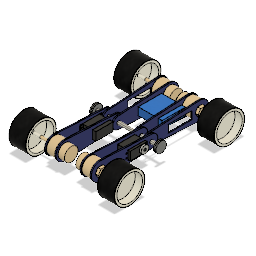
car v16 (Autodesk Fusion 360 design; units mm, degrees)
Autodesk Fusion 360 part; units mm, degrees
sketch "Sketch1" plane through (0, 0, 0) normal (0, 0, 1) x (1, 0, 0) in component "far_leg"
  circle A0 centre (0, 0) radius 6.5
  line L0 (0, 0) -> (120, 0)
  circle A1 centre (120, 0) radius 4
  line L1 (1.225, 20.9642) -> (120.8167, 13.9762)
  line L2 (1.225, -20.9642) -> (120.8167, -13.9762)
  line L3 (19, 0) -> (19, 9)
  line L4 (19, 9) -> (74, 9)
  line L5 (74, 9) -> (74, -9)
  line L6 (74, -9) -> (19, -9)
  line L7 (19, -9) -> (19, 0)
  arc A2 (1.225, 20.9642) -> (1.225, -20.9642) centre (0, 0) ccw
  arc A3 (120.8167, -13.9762) -> (120.8167, 13.9762) centre (120, 0) ccw
  dimension "d1" = 13
  dimension "d2" = 120
  dimension "d3" = 8
  dimension "d4" = 42
  dimension "d5" = 28
  dimension "d183" = 19
  dimension "d184" = 9
  dimension "d186" = 55
  dimension "d187" = 18
  dimension "d188" = 55
  dimension "d272" = 9
  constraint coincident A0.centre L0.start
  constraint horizontal L0
  constraint coincident L0.end A1.centre
  constraint concentric A1 A3
  constraint tangent L1 A3
  constraint tangent L2 A3
  constraint tangent L1 A2
  constraint tangent L2 A2
  constraint perpendicular L0 L3
  constraint perpendicular L3 L4
  constraint perpendicular L0 L5
  constraint perpendicular L5 L6
  measures "d1" diameter of A0
  measures "d2" distance of A0.centre L0.end
  measures "d3" diameter of A1
  measures "d4" diameter of A2
  measures "d5" diameter of A3
  measures "d183" distance of A0.centre L3.start
  measures "d184" distance of L3.start L3.end
  measures "d186" distance of L3.end L4.end
  measures "d187" distance of L4.end L5.end
  measures "d188" distance of L5.end L6.end
  measures "d272" distance of L0 L4
extrude "Extrude1" add sketch "Sketch1" along normal blind 3 makes body 1 in component "far_leg"
sketch "Sketch1 (2)" plane through (0, 0, 0) normal (0, 0, 1) x (1, 0, 0) in component "motor"
  circle A0 centre (0, 0) radius 16
  dimension "d37" = 32
  constraint coincident A0.centre origin
  measures "d37" diameter of A0
extrude "Extrude1'" add sketch "Sketch1 (2)" along normal blind 18 separate body makes body 2 in component "motor"
sketch "Sketch2" plane through (0, 0, 18) normal (0, 0, 1) x (1, 0, 0) in component "motor"
  circle A0 centre (0, 0) radius 16
  circle A1 centre (0, 0) radius 19
  dimension "d40" = 38
  constraint coincident A0.centre A1.centre
  measures "d40" diameter of A1
extrude "Extrude2" add sketch "Sketch2" along normal blind 21 contours A0 | A1 bodies 2 in component "motor"
sketch "Sketch3" plane through (0, 0, 39) normal (0, 0, 1) x (1, 0, 0) in component "motor"
  circle A0 centre (0, 0) radius 19
  line L0 (5.75, -9.9593) -> (11.5, 0)
  line L1 (11.5, 0) -> (5.75, 9.9593)
  line L2 (5.75, 9.9593) -> (-5.75, 9.9593)
  line L3 (-5.75, 9.9593) -> (-11.5, 0)
  line L4 (-11.5, 0) -> (-5.75, -9.9593)
  line L5 (-5.75, -9.9593) -> (5.75, -9.9593)
  line L6 (0, 0) -> (29.7634, 0) construction
  dimension "d43" = 11.5
  constraint coincident A0.centre L6.start
  constraint horizontal L6
  constraint parallel L2 L6
  measures "d43" distance of L0.start A0.centre
extrude "Extrude3" add sketch "Sketch3" along normal blind 10 and the other way blind -3 separate body contours L0 L1 L2 L3 L4 L5 makes body 3 in component "motor"
sketch "Sketch4" plane through (0, 0, 49) normal (0, 0, 1) x (1, 0, 0) in component "motor"
  line L0 (-5.75, -9.9593) -> (5.75, -9.9593)
  line L1 (5.75, -9.9593) -> (11.5, 0)
  line L2 (11.5, 0) -> (5.75, 9.9593)
  line L3 (5.75, 9.9593) -> (-5.75, 9.9593)
  line L4 (-5.75, 9.9593) -> (-11.5, 0)
  line L5 (-11.5, 0) -> (-5.75, -9.9593)
  circle A0 centre (0, 0) radius 3
  dimension "d46" = 6
  constraint coincident A0.centre origin
  measures "d46" diameter of A0
extrude "Extrude4" add sketch "Sketch4" along normal blind 22 and the other way up to surface (10 mm away) contours A0 bodies 3 2 in component "motor"
sketch "Sketch1 (3)" plane through (0, 0, 0) normal (0, 0, 1) x (1, 0, 0) in component "wheel"
  circle A0 centre (0, 0) radius 35
  circle A1 centre (0, 0) radius 30
  dimension "d49" = 70
  dimension "d50" = 60
  constraint coincident A0.centre A1.centre
  measures "d49" diameter of A0
  measures "d50" diameter of A1
extrude "Extrude1''" add sketch "Sketch1 (3)" along normal mid plane 40 separate body makes body 4 in component "wheel"
sketch "Sketch2 (2)" plane through (0, 0, 0) normal (0, 0, 1) x (1, 0, 0) in component "wheel"
  circle A0 centre (0, 0) radius 30
  dimension "d53" = 60
  constraint coincident A0.centre origin
  measures "d53" diameter of A0
extrude "Extrude2'" add sketch "Sketch2 (2)" along normal mid plane 6 bodies 4 in component "wheel"
sketch "Sketch3 (2)" plane through (0, 0, -3) normal (0, 0, -1) x (-1, 0, 0) in component "wheel"
  circle A0 centre (0, 0) radius 30
  circle A1 centre (0, 0) radius 3
  dimension "d56" = 6
  constraint coincident A0.centre A1.centre
  measures "d56" diameter of A1
extrude "Extrude3'" add sketch "Sketch3 (2)" along normal blind 17 contours A1 bodies 4 in component "wheel"
sketch "Sketch1 (4)" plane through (0, 0, 0) normal (0, 0, 1) x (1, 0, 0) in component "tyre"
  circle A0 centre (0, 0) radius 35
  circle A1 centre (0, 0) radius 36
  dimension "d68" = 70
  dimension "d69" = 72
  constraint coincident A0.centre A1.centre
  constraint concentric A0 A1
  measures "d68" diameter of A0
  measures "d69" diameter of A1
extrude "Extrude1'''" add sketch "Sketch1 (4)" along normal mid plane 40 separate body makes body 5 in component "tyre"
move_body "Move1" bodies 4 to x (0, 0, 1) y (0, 1, 0) z (-1, 0, 0) at (44, 0, -196) in component "wheel"
move_body "Move1'" bodies 3 to x (0, 0, 1) y (0, 1, 0) z (-1, 0, 0) at (135, 0, -105) in component "motor"
move_body "Move1''" bodies 1 to x (0, 0, 1) y (0, 1, 0) z (-1, 0, 0) at (96, 0, -144) in component "far_leg"
move_body "Move1'''" bodies 5 to x (0, 0, 1) y (0, 1, 0) z (-1, 0, 0) at (44, 0, -196) in component "tyre"
sketch "Sketch1 (5)" plane through (0, 0, 0) normal (1, 0, 0) x (0, 0, -1) in component "axle"
  circle A0 centre (0, 0) radius 4
  dimension "d156" = 8
  constraint coincident A0.centre origin
  measures "d156" diameter of A0
extrude "Extrude1''''" add sketch "Sketch1 (5)" along normal blind 150 separate body makes body 6 in component "axle"
sketch "Sketch1 (6)" plane through (0, 0, 0) normal (1, 0, 0) x (0, 0, -1) in component "front_far_leg"
  circle A0 centre (0, 0) radius 4
  line L0 (0, 0) -> (-132.6267, 0) construction
  line L1 (0, 0) -> (0, 16.3072) construction
  line L2 (0, 0) -> (0, -19.0636) construction
  circle A1 centre (-120, 0) radius 6.5
  line L3 (-15, 10) -> (-55, 10)
  line L4 (-55, 10) -> (-55, -10)
  line L5 (-55, -10) -> (-15, -10)
  line L6 (-15, -10) -> (-15, 10)
  line L7 (0, 15) -> (-118.9467, 20.9736)
  line L8 (0, -15) -> (-118.9467, -20.9736)
  arc A2 (-118.9467, 20.9736) -> (-118.9467, -20.9736) centre (-120, 0) ccw
  arc A3 (0, -15) -> (0, 15) centre (0, 0) ccw
  line L9 (-15, 5) -> (-11, 5) construction
  line L10 (-15, -5) -> (-11, -5) construction
  line L11 (-55, 5) -> (-59, 5) construction
  line L12 (-55, -5) -> (-59, -5) construction
  circle A4 centre (-11, 5) radius 1.5
  circle A5 centre (-11, -5) radius 1.5
  circle A6 centre (-59, 5) radius 1.5
  circle A7 centre (-59, -5) radius 1.5
  dimension "d288" = 8
  dimension "d289" = 30
  dimension "d290" = 13
  dimension "d291" = 42
  dimension "d292" = 120
  dimension "d293" = 40
  dimension "d294" = 20
  dimension "d295" = 10
  dimension "d296" = 15
  dimension "d398" = 4
  dimension "d399" = 4
  dimension "d400" = 4
  dimension "d401" = 4
  dimension "d402" = 5
  dimension "d403" = 5
  dimension "d404" = 5
  dimension "d405" = 5
  dimension "d406" = 3
  dimension "d407" = 3
  dimension "d408" = 3
  dimension "d409" = 3
  constraint coincident A0.centre L0.start
  constraint concentric A0 A3
  constraint horizontal L0
  constraint perpendicular L0 L1
  constraint perpendicular L0 L2
  constraint coincident L0 A1.centre
  constraint concentric A1 A2
  constraint horizontal L3
  constraint vertical L4
  constraint horizontal L5
  constraint vertical L6
  constraint coincident L1 L7.start
  constraint tangent L7 A2
  constraint coincident L2 L8.start
  constraint tangent L8 A2
  constraint coincident L6 L9.start
  constraint perpendicular L6 L9
  constraint coincident L6 L10.start
  constraint perpendicular L6 L10
  constraint coincident L4 L11.start
  constraint perpendicular L4 L11
  constraint coincident L4 L12.start
  constraint perpendicular L4 L12
  constraint coincident L9.end A4.centre
  constraint coincident L10.end A5.centre
  constraint coincident L11.end A6.centre
  constraint coincident L12.end A7.centre
  measures "d288" diameter of A0
  measures "d289" diameter of A3
  measures "d290" diameter of A1
  measures "d291" diameter of A2
  measures "d292" distance of A0.centre A1.centre
  measures "d293" distance of L3.start L3.end
  measures "d294" distance of L3.start L5.end
  measures "d295" distance of L0 L3
  measures "d296" distance of L2 L6
  measures "d398" distance of L9.start L9.end
  measures "d399" distance of L10.start L10.end
  measures "d400" distance of L11.start L11.end
  measures "d401" distance of L12.start L12.end
  measures "d402" distance of L0 L9
  measures "d403" distance of L0 L10
  measures "d404" distance of L0 L11
  measures "d405" distance of L0 L12
  measures "d406" diameter of A4
  measures "d407" diameter of A5
  measures "d408" diameter of A6
  measures "d409" diameter of A7
extrude "Extrude1'''''" add sketch "Sketch1 (6)" along normal blind 3 separate body makes body 7 in component "front_far_leg"
sketch "Sketch1 (7)" plane through (0, 0, 0) normal (1, 0, 0) x (0, 0, -1) in component "front_mid_leg"
  line L0 (-15, -10) -> (-15, 10)
  line L1 (0, 0) -> (-150, 0) construction
  circle A0 centre (-120, 0) radius 16
  line L2 (-55, -10) -> (-15, -10)
  line L3 (0, 0) -> (0, 25.1671) construction
  line L4 (-55, 10) -> (-55, -10)
  line L5 (0, 15) -> (-118.9467, 20.9736)
  line L6 (-15, 10) -> (-55, 10)
  line L7 (0, -15) -> (-118.9467, -20.9736)
  circle A1 centre (0, 0) radius 4
  line L8 (0, 0) -> (0, 72.997) construction
  arc A2 (0, -15) -> (0, 15) centre (0, 0) ccw
  arc A3 (-118.9467, 20.9736) -> (-118.9467, -20.9736) centre (-120, 0) ccw
  dimension "d309" = 8
  dimension "d310" = 30
  dimension "d311" = 32
  dimension "d312" = 42
  dimension "d313" = 120
  dimension "d314" = 150
  dimension "d315" = 40
  dimension "d316" = 20
  dimension "d317" = 10
  dimension "d318" = 15
  constraint coincident L1.start L3.start
  constraint horizontal L1
  constraint perpendicular L1 L8
  constraint perpendicular L1 L3
  constraint coincident A0.centre L1
  constraint concentric A0 A3
  constraint horizontal L6
  constraint vertical L4
  constraint horizontal L2
  constraint vertical L0
  constraint coincident L5.start L8
  constraint tangent L5 A3
  constraint coincident L7.start L3
  constraint tangent L7 A3
  measures "d309" diameter of A1
  measures "d310" diameter of A2
  measures "d311" diameter of A0
  measures "d312" diameter of A3
  measures "d313" distance of A0.centre L1.start
  measures "d314" distance of L1.start L1.end
  measures "d315" distance of L0.end L4.start
  measures "d316" distance of L0.start L0.end
  measures "d317" distance of L1 L6
  measures "d318" distance of L0 L3
extrude "Extrude1''''''" add sketch "Sketch1 (7)" along normal blind 3 separate body makes body 8 in component "front_mid_leg"
sketch "Sketch5" plane through (0, 0, 0) normal (1, 0, 0) x (0, 0, -1)
sketch "Sketch1 (8)" plane through (0, 0, 0) normal (1, 0, 0) x (0, 0, -1) in component "rear_mid_leg"
  circle A0 centre (0, 0) radius 16
  line L0 (-19, 9) -> (-74, 9)
  line L1 (-74, 9) -> (-74, -9)
  line L2 (-74, -9) -> (-19, -9)
  line L3 (-19, -9) -> (-19, 9)
  line L4 (0, 0) -> (-87.4504, 0) construction
  circle A1 centre (-120, 0) radius 4
  line L5 (-1.225, 20.9642) -> (-120.8167, 13.9762)
  line L6 (-120.8167, -13.9762) -> (-1.225, -20.9642)
  arc A2 (-1.225, -20.9642) -> (-1.225, 20.9642) centre (0, 0) ccw
  arc A3 (-120.8167, 13.9762) -> (-120.8167, -13.9762) centre (-120, 0) ccw
  dimension "d337" = 32
  dimension "d339" = 55
  dimension "d340" = 18
  dimension "d341" = 9
  dimension "d342" = 19
  dimension "d343" = 8
  dimension "d344" = 28
  dimension "d345" = 120
  constraint coincident A0.centre L4.start
  constraint horizontal L0
  constraint vertical L1
  constraint horizontal L2
  constraint vertical L3
  constraint horizontal L4
  constraint coincident L4 A1.centre
  constraint concentric A1 A3
  constraint tangent L5 A3
  constraint tangent L6 A3
  measures "d337" diameter of A0
  measures "d339" distance of L0.start L0.end
  measures "d340" distance of L0.start L2.end
  measures "d341" distance of L0 L4
  measures "d342" distance of A0.centre L3
  measures "d343" diameter of A1
  measures "d344" diameter of A3
  measures "d345" distance of A1.centre A0.centre
extrude "Extrude1'''''''" add sketch "Sketch1 (8)" along normal blind 3 separate body makes body 9 in component "rear_mid_leg"
sketch "Sketch1 (9)" plane through (0, 0, 0) normal (0, 1, 0) x (1, 0, 0) in component "battery"
  line L0 (9, 27.5) -> (-9, 27.5)
  line L1 (-9, 27.5) -> (-9, -27.5)
  line L2 (-9, -27.5) -> (9, -27.5)
  line L3 (9, -27.5) -> (9, 27.5)
  line L4 (9, 27.5) -> (-9, -27.5) construction
  line L5 (-9, 27.5) -> (9, -27.5) construction
  dimension "d390" = 18
  dimension "d391" = 55
  constraint horizontal L0
  constraint perpendicular L0 L1
  constraint parallel L0 L2
  constraint parallel L1 L3
  constraint coincident L4 origin
  constraint coincident L5 origin
  measures "d390" distance of L1.end L2.end
  measures "d391" distance of L0.end L1.end
extrude "Extrude1''''''''" add sketch "Sketch1 (9)" along normal blind 68 separate body makes body 10 in component "battery"
sketch "Sketch1 (10)" plane through (0, 0, 0) normal (0, 1, 0) x (1, 0, 0) in component "servo"
  line L0 (0, 0) -> (40, 0)
  line L1 (40, 0) -> (40, -40)
  line L2 (40, -40) -> (0, -40)
  line L3 (0, -40) -> (0, 0)
  dimension "d410" = 40
  dimension "d411" = 40
  constraint horizontal L0
  constraint vertical L1
  constraint horizontal L2
  constraint vertical L3
  constraint coincident L0.start L3.end
  measures "d410" distance of L0.start L0.end
  measures "d411" distance of L0.start L2.end
extrude "Extrude1'''''''''" add sketch "Sketch1 (10)" along normal blind 20 separate body makes body 11 in component "servo"
sketch "Sketch2 (3)" plane through (0, 0, 0) normal (-1, 0, 0) x (0, 0, 1) in component "servo"
  line L0 (0, 0) -> (40, 0)
  line L1 (40, 0) -> (40, 20)
  line L2 (40, 20) -> (0, 20)
  line L3 (0, 20) -> (0, 0)
  line L4 (0, 20) -> (-6, 20)
  line L5 (-6, 20) -> (-6, 0)
  line L6 (-6, 0) -> (0, 0)
  line L7 (0, 0) -> (0, 20)
  line L8 (0, 15) -> (-4, 15) construction
  circle A0 centre (-4, 15) radius 1.5
  line L9 (0, 5) -> (-4, 5) construction
  circle A1 centre (-4, 5) radius 1.5
  line L10 (40, 20) -> (46, 20)
  line L11 (46, 20) -> (46, 0)
  line L12 (46, 0) -> (40, 0)
  line L13 (40, 0) -> (40, 20)
  line L14 (40, 15) -> (44, 15) construction
  line L15 (40, 5) -> (44, 5) construction
  circle A2 centre (44, 15) radius 1.5
  circle A3 centre (44, 5) radius 1.5
  dimension "d414" = 6
  dimension "d415" = 4
  dimension "d416" = 5
  dimension "d417" = 3
  dimension "d418" = 4
  dimension "d419" = 5
  dimension "d420" = 3
  dimension "d421" = 6
  dimension "d422" = 20
  dimension "d423" = 4
  dimension "d424" = 4
  dimension "d425" = 5
  dimension "d426" = 5
  dimension "d427" = 3
  dimension "d428" = 3
  constraint horizontal L4
  constraint vertical L5
  constraint horizontal L6
  constraint vertical L7
  constraint coincident L2.end L3.start
  constraint coincident L0.start L6
  constraint coincident L7 L8.start
  constraint perpendicular L7 L8
  constraint coincident L8.end A0.centre
  constraint coincident L3 L9.start
  constraint perpendicular L3 L9
  constraint coincident L9.end A1.centre
  constraint horizontal L10
  constraint vertical L11
  constraint horizontal L12
  constraint vertical L13
  constraint coincident L1.end L2.start
  constraint coincident L13 L14.start
  constraint perpendicular L13 L14
  constraint coincident L1 L15.start
  constraint perpendicular L1 L15
  constraint coincident L14.end A2.centre
  constraint coincident L15.end A3.centre
  measures "d414" distance of L2.end L4.end
  measures "d415" distance of L8.start L8.end
  measures "d416" distance of L4 L8
  measures "d417" diameter of A0
  measures "d418" distance of L9.start L9.end
  measures "d419" distance of L6 L9
  measures "d420" diameter of A1
  measures "d421" distance of L1.end L10.end
  measures "d422" distance of L1.end L0.end
  measures "d423" distance of L14.start L14.end
  measures "d424" distance of L15.start L15.end
  measures "d425" distance of L10 L14
  measures "d426" distance of L12 L15
  measures "d427" diameter of A2
  measures "d428" diameter of A3
extrude "Extrude2''" add sketch "Sketch2 (3)" along normal blind -10 and the other way blind 8 contours L3 L4 L5 L6 L7 | L1 L10 L11 L12 L13 bodies 11 in component "servo"
sketch "Sketch3 (3)" plane through (0, 0, 0) normal (-1, 0, 0) x (0, 0, 1) in component "servo"
  line L0 (0, 0) -> (40, 0)
  line L1 (40, 0) -> (40, 20)
  line L2 (40, 20) -> (0, 20)
  line L3 (0, 20) -> (0, 0)
  line L4 (0, 10) -> (50.7597, 10) construction
  circle A0 centre (9, 10) radius 3
  dimension "d433" = 6
  dimension "d434" = 9
  constraint midpoint L3 L4.start
  constraint perpendicular L3 L4
  constraint coincident L4 A0.centre
  measures "d433" diameter of A0
  measures "d434" distance of L3 A0.centre
extrude "Extrude3''" add sketch "Sketch3 (3)" along normal blind 4 contours A0 bodies 11 in component "servo"
sketch "Sketch1 (11)" plane through (0, 0, 0) normal (-1, 0, 0) x (0, 0, 1) in component "Component"
  circle A0 centre (9, 10) radius 3
  line L0 (0, 0) -> (40, 0)
  line L1 (40, 0) -> (40, 20)
  line L2 (40, 20) -> (0, 20)
  line L3 (0, 20) -> (0, 0)
  circle A1 centre (9, 10) radius 3
  circle A2 centre (9, 10) radius 9
  dimension "d437" = 6
  dimension "d438" = 18
  constraint coincident A0.centre A1.centre
  constraint concentric A1 A2
  measures "d437" diameter of A1
  measures "d438" diameter of A2
extrude "Extrude1''''''''''" add sketch "Sketch1 (11)" along normal blind 4 separate body contours A2 makes body 12 in component "Component"
sketch "Sketch1 (12)" plane through (0, 0, 0) normal (1, 0, 0) x (0, 0, -1) in component "name"
  circle A0 centre (0, 0) radius 4
  circle A1 centre (0, 0) radius 12.5
  dimension "d472" = 8
  dimension "d473" = 25
  constraint coincident A0.centre A1.centre
  constraint concentric A0 A1
  measures "d472" diameter of A0
  measures "d473" diameter of A1
extrude "Extrude1'''''''''''" add sketch "Sketch1 (12)" along normal blind 3 separate body makes body 13 in component "name"
sketch "Sketch1 (13)" plane through (0, 0, 0) normal (-1, 0, 0) x (0, 0, 1) in component "Component'"
  circle A0 centre (0, 0) radius 4
  circle A1 centre (0, 0) radius 12.5
  circle A2 centre (0, 0) radius 12.5
  dimension "d476" = 25
  constraint coincident A0.centre A1.centre
  measures "d476" diameter of A2
extrude "Extrude1''''''''''''" add sketch "Sketch1 (13)" along normal blind 3 separate body contours A0 | A1 A2 makes body 14 in component "Component'"
component "far_leg" placed x (1, 0, 0) y (0, 1, 0) z (0, 0, 1) at (-139.5928, 42.0832, 28.8359)
component "motor" placed x (1, 0, 0) y (0, 1, 0) z (0, 0, 1) at (-139.5928, 42.0832, -10.1641)
component "wheel" placed x (1, 0, 0) y (0, 1, 0) z (0, 0, 1) at (-139.5928, 42.0832, 80.8359)
component "far_leg" placed x (1, 0, 0) y (0, 1, 0) z (0, 0, 1) at (-44.5928, 42.0832, 28.8359)
component "motor" placed x (-1, 0, 0) y (0, -1, 0) z (0, 0, 1) at (144.4072, 42.0832, -10.1641)
component "wheel" placed x (-1, 0, 0) y (0, -1, 0) z (0, 0, 1) at (144.4072, 42.0832, 80.8359)
component "axle" placed x (1, 0, 0) y (0, 1, 0) z (0, 0, 1) at (-72.5928, 42.0832, 4.8359)
component "wheel" placed x (1, 0, 0) y (0, 1, 0) z (0, 0, 1) at (-145.5928, 42.0832, 320.8359)
component "wheel" placed x (-1, 0, 0) y (0, -1, 0) z (0, 0, 1) at (150.4072, 42.0832, 320.8359)
component "motor" placed x (1, 0, 0) y (0, 1, 0) z (0, 0, 1) at (-145.5928, 42.0832, 229.8359)
component "motor" placed x (-1, 0, 0) y (0, -1, 0) z (0, 0, 1) at (150.4072, 42.0832, 229.8359)
component "front_far_leg" placed x (1, 0, 0) y (0, 1, 0) z (0, 0, 1) at (-52.5928, 42.0832, 4.8359)
component "front_mid_leg" placed x (1, 0, 0) y (0, 1, 0) z (0, 0, 1) at (-28.5928, 42.0832, 4.8359)
component "rear_mid_leg" placed x (1, 0, 0) y (0, 1, 0) z (0, 0, 1) at (-22.5928, 42.0832, -115.1641)
component "rear_mid_leg" placed x (1, 0, 0) y (0, 1, 0) z (0, 0, 1) at (24.4072, 42.0832, -115.1641)
component "battery" placed x (0, 1, 0) y (-1, 0, 0) z (0, 0, 1) at (36.4072, 42.0832, -68.6641)
component "servo" placed x (1, 0, 0) y (0, 1, 0) z (0, 0, 1) at (-57.5928, 32.0832, 19.8359)
component "front_mid_leg" placed x (1, 0, 0) y (0, 1, 0) z (0, 0, 1) at (30.4072, 42.0832, 4.8359)
component "front_far_leg" placed x (1, 0, 0) y (0, 1, 0) z (0, 0, 1) at (54.4072, 42.0832, 4.8359)
component "servo" placed x (-1, 0, 0) y (0, -1, 0) z (0, 0, 1) at (62.4072, 52.0832, 19.8359)
component "name" placed x (1, 0, 0) y (0, 1, 0) z (0, 0, 1) at (-72.5928, 42.0832, 4.8359)
component "name" placed x (-1, 0, 0) y (0, -1, 0) z (0, 0, 1) at (77.4072, 42.0832, 4.8359)
component "tyre" placed x (1, 0, 0) y (0, 1, 0) z (0, 0, 1) at (0, 0, 0) in component "wheel"
component "Component" placed x (1, 0, 0) y (0, 1, 0) z (0, 0, 1) at (0, 0, 0) in component "servo"
component "Component'" placed x (1, 0, 0) y (0, 1, 0) z (0, 0, 1) at (0, 0, 0) in component "name"
